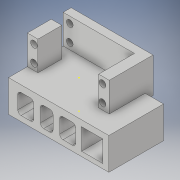
# Autodesk Inventor part: Nov 21 holder for arm server (resized hole)
Saved by Autodesk Inventor 2018 (Build 220112000, 112)
## iProperties
Created: 2017-11-08
Part Number: Nov 21 holder for arm server (resized hole)
Material: Generic
Document SubType Name: Modeling
Designer: battin.michael
Density: 1 g/cm^3
Appearance: Default
Author: battin.michael
Autodesk Inventor part; units mm, degrees
ref_plane "YZ Plane" through (0, 0, 0) normal (1, 0, 0) x (0, 1, 0)
ref_plane "XZ Plane" through (0, 0, 0) normal (0, 1, 0) x (-1, 0, 0)
ref_plane "XY Plane" through (0, 0, 0) normal (0, 0, 1) x (1, 0, 0)
sketch "Sketch1" plane through (0, 0, 0) normal (0, 1, 0) x (-1, 0, 0)
  line L0 (59.1344, 5.7229) -> (-34.3376, 5.7229)
  line L1 (-34.3376, 5.7229) -> (-34.3376, -46.6011)
  line L2 (-34.3376, -46.6011) -> (59.1344, -46.6011)
  line L3 (59.1344, -46.6011) -> (59.1344, 5.7229)
  point P0 (0, 0)
  dimension "d0" = 52.324
  dimension "d1" = 93.472
  constraints: 8 end point, 2 parallel, 1 horizontal, 1 perpendicular
  measures "d0" distance between parallel lines of L2 L0
  measures "d1" distance between parallel lines of L1 L3
extrude "Extrusion1" add sketch "Sketch1" along normal blind 5.08
sketch "Sketch2" plane through (0, 5.08, 0) normal (0, 1, 0) x (1, 0, 0)
  line L0 (34.3376, -5.7229) -> (34.3376, 46.6011) projected
  line L1 (-59.1344, -5.7229) -> (34.3376, -5.7229) projected
  line L2 (34.3376, 46.6011) -> (27.9876, 46.6011)
  line L3 (27.9876, 46.6011) -> (27.9876, -5.7229)
  line L4 (27.9876, -5.7229) -> (34.3376, -5.7229)
  line L5 (34.3376, -5.7229) -> (34.3376, 46.6011)
  line L6 (8.9376, 46.6011) -> (2.5876, 46.6011)
  line L7 (2.5876, 46.6011) -> (2.5876, -5.7229)
  line L8 (2.5876, -5.7229) -> (8.9376, -5.7229)
  line L9 (8.9376, -5.7229) -> (8.9376, 46.6011)
  line L10 (34.3376, 46.6011) -> (-59.1344, 46.6011) projected
  line L11 (-59.1344, 46.6011) -> (-59.1344, -5.7229) projected
  line L12 (-52.7844, 46.6011) -> (-59.1344, 46.6011)
  line L13 (-59.1344, 46.6011) -> (-59.1344, -5.7229)
  line L14 (-59.1344, -5.7229) -> (-52.7844, -5.7229)
  line L15 (-52.7844, -5.7229) -> (-52.7844, 46.6011)
  point P0 (0, 0)
  dimension "d4" = 6.35
  dimension "d5" = 19.05
  dimension "d6" = 6.35
  dimension "d7" = 6.35
  constraints: 24 end point, 6 parallel, 3 horizontal, 3 perpendicular, 3 point on line
  measures "d4" distance between parallel lines of L0 L3
  measures "d5" distance between parallel lines of L3 L9
  measures "d6" distance between parallel lines of L7 L9
  measures "d7" distance between parallel lines of L13 L15
extrude "Extrusion2" add sketch "Sketch2" along normal blind 19.05 contours L1 L3 L2 L0 | L1 L7 L6 L9 | L1 L11 L10 L15
sketch "Sketch3" plane through (0, 24.13, 0) normal (0, 1, 0) x (1, 0, 0)
  line L0 (34.3376, -5.7229) -> (34.3376, 46.6011) projected
  line L1 (-59.1344, 46.6011) -> (-59.1344, -5.7229) projected
  line L2 (34.3376, 46.6011) -> (-59.1344, 46.6011)
  line L3 (-59.1344, 46.6011) -> (-59.1344, -5.7229)
  line L4 (-59.1344, -5.7229) -> (34.3376, -5.7229)
  line L5 (34.3376, -5.7229) -> (34.3376, 46.6011)
  point P0 (0, 0)
  constraints: 8 end point, 2 parallel, 1 horizontal, 1 perpendicular
extrude "Extrusion3" add sketch "Sketch3" along normal blind 6.35
sketch "Sketch4" plane through (0, 30.48, 0) normal (0, 1, 0) x (1, 0, 0)
  point P0 (0, 0)
sketch "Sketch5" plane through (0, 30.48, 0) normal (0, 1, 0) x (1, 0, 0)
  line L0 (-59.1344, -5.7229) -> (34.3376, -5.7229) projected
  line L1 (-59.1344, -5.7229) -> (-51.5144, -5.7229)
  line L2 (-51.5144, -5.7229) -> (-51.5144, 46.6011)
  line L3 (-51.5144, 46.6011) -> (-59.1344, 46.6011)
  line L4 (-59.1344, 46.6011) -> (-59.1344, -5.7229)
  line L5 (-52.7844, -5.7229) -> (2.5876, -5.7229) projected
  line L6 (6.5246, -5.7229) -> (14.1446, -5.7229)
  line L7 (14.1446, -5.7229) -> (14.1446, 46.6011)
  line L8 (14.1446, 46.6011) -> (6.5246, 46.6011)
  line L9 (6.5246, 46.6011) -> (6.5246, -5.7229)
  point P0 (0, 0)
  dimension "d12" = 7.62
  dimension "d13" = 7.62
  dimension "d14" = 58.039
  constraints: 16 end point, 4 parallel, 2 horizontal, 2 perpendicular, 1 point on line
  measures "d12" distance of L3.end L2.end
  measures "d13" distance of L8.end L7.end
  measures "d14" distance between parallel lines of L9 L2
extrude "Extrusion4" add sketch "Sketch5" along normal blind 27.94
sketch "Sketch6" plane through (0, 58.42, 0) normal (0, 1, 0) x (1, 0, 0)
  point P0 (0, 0)
sketch "Sketch7" plane through (0, 58.42, 0) normal (0, 1, 0) x (1, 0, 0)
  line L0 (-59.1344, -5.7229) -> (-51.5144, -5.7229) projected
  line L1 (-51.5144, -5.7229) -> (-51.5144, 46.6011) projected
  line L2 (-59.1344, -5.7229) -> (-51.5144, -5.7229)
  line L3 (-51.5144, -5.7229) -> (-51.5144, 12.3111)
  line L4 (-51.5144, 12.3111) -> (-59.1344, 12.3111)
  line L5 (-59.1344, 12.3111) -> (-59.1344, -5.7229)
  line L6 (6.5246, -5.7229) -> (6.5246, 46.6011) projected
  line L7 (14.1446, -5.7229) -> (14.1446, 46.6011) projected
  line L8 (6.5246, -5.7229) -> (14.1446, -5.7229)
  line L9 (14.1446, -5.7229) -> (14.1446, 12.3111)
  line L10 (14.1446, 12.3111) -> (6.5246, 12.3111)
  line L11 (6.5246, 12.3111) -> (6.5246, -5.7229)
  point P0 (0, 0)
  dimension "d17" = 18.034
  constraints: 16 end point, 4 parallel, 2 horizontal, 2 perpendicular, 2 point on line
  measures "d17" distance between parallel lines of L4 L0
extrude "Extrusion5" cut sketch "Sketch7" against normal blind 27.94
sketch "Sketch8" plane through (0, 58.42, 0) normal (0, 1, 0) x (1, 0, 0)
  line L0 (34.3376, 46.6011) -> (-59.1344, 46.6011) projected
  line L1 (-51.5144, 46.6011) -> (-51.5144, 12.3111) projected
  line L2 (-59.1344, 46.6011) -> (-51.5144, 46.6011)
  line L3 (-51.5144, 46.6011) -> (-51.5144, 35.1711)
  line L4 (-51.5144, 35.1711) -> (-59.1344, 35.1711)
  line L5 (-59.1344, 35.1711) -> (-59.1344, 46.6011)
  point P0 (0, 0)
  dimension "d20" = 11.43
  constraints: 8 end point, 2 parallel, 1 horizontal, 1 perpendicular, 1 point on line
  measures "d20" distance between parallel lines of L4 L0
extrude "Extrusion6" cut sketch "Sketch8" against normal blind 27.94
sketch "Sketch9" plane through (34.3376, 0, -46.6011) normal (0, 0, -1) x (-1, 0, 0)
  line L0 (93.472, 30.48) -> (0, 30.48) projected
  line L1 (27.813, 30.48) -> (20.193, 30.48) projected
  line L2 (93.472, 30.48) -> (20.193, 30.48)
  line L3 (20.193, 30.48) -> (20.193, 24.13)
  line L4 (6.35, 24.13) -> (25.4, 24.13) projected
  line L5 (31.75, 24.13) -> (87.122, 24.13) projected
  line L6 (25.4, 24.13) -> (31.75, 24.13)
  line L7 (87.122, 5.08) -> (87.122, 24.13) projected
  line L8 (31.75, 24.13) -> (87.122, 24.13)
  line L9 (93.472, 0) -> (93.472, 30.48) projected
  line L10 (87.122, 24.13) -> (93.472, 24.13)
  point P0 (34.3376, 0)
  constraints: 10 end point, 3 point on line, 2 horizontal, 2 perpendicular
extrude "Extrusion7" add sketch "Sketch9" along normal blind 7.62
sketch "Sketch10" plane through (0, 30.48, 0) normal (0, 1, 0) x (1, 0, 0)
  line L0 (14.1446, 46.6011) -> (14.1446, 54.2211) projected
  line L1 (-59.1344, 54.2211) -> (14.1446, 54.2211) projected
  line L2 (14.1446, 46.6011) -> (-59.1344, 46.6011)
  line L3 (-59.1344, 46.6011) -> (-59.1344, 54.2211)
  line L4 (-59.1344, 54.2211) -> (14.1446, 54.2211)
  line L5 (14.1446, 54.2211) -> (14.1446, 46.6011)
  point P0 (0, 0)
  constraints: 8 end point, 2 parallel, 1 horizontal, 1 perpendicular
extrude "Extrusion8" add sketch "Sketch10" along normal blind 27.94
fillet "Fillet1" radius 3.175 4 edges at (2.5876, 5.08, -20.4391) (-52.7844, 5.08, -20.4391) (2.5876, 24.13, -20.4391) (-52.7844, 24.13, -20.4391)
sketch "Sketch11" plane through (-59.1344, 58.42, -12.3111) normal (0, 0, 1) x (1, 0, 0)
  point P0 (59.1344, -58.42)
sketch "Sketch12" plane through (-59.1344, 58.42, -12.3111) normal (0, 0, 1) x (1, 0, 0)
  circle A0 centre (3.81, -6.096) radius 2.54
  line L0 (0, 0) -> (7.62, 0) projected
  line L1 (0, -27.94) -> (0, 0) projected
  circle A1 centre (3.81, -21.844) radius 2.54
  line L2 (0, -27.94) -> (7.62, -27.94) projected
  circle A2 centre (69.469, -6.096) radius 2.54
  line L3 (65.659, 0) -> (73.279, 0) projected
  line L4 (73.279, 0) -> (73.279, -27.94) projected
  circle A3 centre (69.469, -21.844) radius 2.54
  line L5 (0, -27.94) -> (93.472, -27.94) projected
  point P0 (59.1344, -58.42)
  dimension "d29" = 6.096
  dimension "d30" = 3.81
  dimension "d31" = 5.08
  dimension "d32" = 5.08
  dimension "d33" = 3.81
  dimension "d34" = 6.096
  dimension "d35" = 5.08
  dimension "d36" = 6.096
  dimension "d37" = 3.81
  dimension "d38" = 5.08
  dimension "d39" = 3.81
  dimension "d40" = 6.096
  constraints: 4 centre point
  measures "d29" distance from line of L0 A0.centre
  measures "d30" distance from line of L1 A0.centre
  measures "d31" diameter of A0
  measures "d32" diameter of A1
  measures "d33" distance from line of A1.centre L1
  measures "d34" distance from line of L2 A1.centre
  measures "d35" diameter of A2
  measures "d36" distance from line of A2.centre L3
  measures "d37" distance from line of A2.centre L4
  measures "d38" diameter of A3
  measures "d39" distance from line of A3.centre L4
  measures "d40" distance from line of L5 A3.centre
hole "Hole1" at (-55.3244, 52.324, -12.3111) at (-55.3244, 36.576, -12.3111) at (10.3346, 52.324, -12.3111) at (10.3346, 36.576, -12.3111) direction (0, 0, -1) diameter 6.35 end through all
sketch "Sketch13" plane through (-59.1344, 0, -46.6011) normal (-1, 0, 0) x (0, 0, 1)
  line L0 (-7.62, 24.13) -> (-7.62, 58.42) projected
  line L1 (-7.62, 58.42) -> (-7.62, 24.13)
  line L2 (0, 24.13) -> (-7.62, 24.13) projected
  line L3 (-7.62, 24.13) -> (0, 24.13)
  line L4 (0, 0) -> (0, 24.13) projected
  line L5 (0, 24.13) -> (0, 0)
  line L6 (0, 0) -> (52.324, 0) projected
  line L7 (0, 0) -> (52.324, 0)
  line L8 (52.324, 0) -> (52.324, 30.48) projected
  line L9 (52.324, 0) -> (52.324, 30.48)
  line L10 (34.29, 30.48) -> (34.29, 58.42) projected
  line L11 (52.324, 30.48) -> (34.29, 30.48)
  line L12 (34.29, 30.48) -> (34.29, 58.42)
  line L13 (34.29, 58.42) -> (11.43, 58.42) projected
  line L14 (34.29, 58.42) -> (11.43, 58.42)
  line L15 (11.43, 30.48) -> (11.43, 58.42) projected
  line L16 (11.43, 58.42) -> (11.43, 30.48)
  line L17 (11.43, 30.48) -> (0, 30.48) projected
  line L18 (11.43, 30.48) -> (0, 30.48)
  line L19 (0, 30.48) -> (0, 58.42) projected
  line L20 (0, 30.48) -> (0, 58.42)
  line L21 (34.29, 58.42) -> (-7.62, 58.42) projected
  line L22 (0, 58.42) -> (-7.62, 58.42)
  point P0 (46.6011, 0)
  constraints: 24 end point, 6 collinear, 3 perpendicular, 1 horizontal, 1 vertical
extrude "Extrusion9" add sketch "Sketch13" along normal blind 2.54 contours L0 L21 L19 L17 L15 L13 L10 L11 L8 L6 L4 L2
sketch "Sketch14" plane through (14.1446, 24.13, -46.6011) normal (1, 0, 0) x (0, 0, -1)
  line L0 (-34.29, 34.29) -> (7.62, 34.29) projected
  line L1 (7.62, 0) -> (7.62, 34.29) projected
  line L2 (-34.29, 34.29) -> (7.62, 34.29)
  line L3 (7.62, 34.29) -> (7.62, 0)
  line L4 (7.62, 0) -> (-34.29, 0)
  line L5 (-34.29, 0) -> (-34.29, 34.29)
  line L6 (0, 0) -> (7.62, 0) projected
  line L7 (0, 6.35) -> (-34.29, 6.35) projected
  line L8 (0, 0) -> (-34.29, 0)
  line L9 (-34.29, 0) -> (-34.29, 6.35)
  line L10 (-34.29, 6.35) -> (0, 6.35)
  line L11 (0, 6.35) -> (0, 0)
  point P0 (-46.6011, -24.13)
  constraints: 16 end point, 4 parallel, 2 horizontal, 2 perpendicular
extrude "Extrusion10" add sketch "Sketch14" along normal blind 2.54 contours L0 L1 L4 L11 L7 L5
sketch "Sketch15" plane through (0, 5.08, 0) normal (0, 1, 0) x (1, 0, 0)
  point P0 (0, 0)
sketch "Sketch16" plane through (0, 5.08, 0) normal (0, 1, 0) x (1, 0, 0)
  line L0 (34.3376, 46.6011) -> (-61.6744, 46.6011) projected
  line L1 (-61.6744, -5.7229) -> (34.3376, -5.7229) projected
  line L2 (-37.502, 46.6011) -> (-31.152, 46.6011)
  line L3 (-31.152, 46.6011) -> (-31.152, -5.7229)
  line L4 (-31.152, -5.7229) -> (-37.502, -5.7229)
  line L5 (-37.502, -5.7229) -> (-37.502, 46.6011)
  line L6 (-19.0447, -5.7229) -> (-12.6947, -5.7229)
  line L7 (-12.6947, -5.7229) -> (-12.6947, 46.6011)
  line L8 (-12.6947, 46.6011) -> (-19.0447, 46.6011)
  line L9 (-19.0447, 46.6011) -> (-19.0447, -5.7229)
  line L10 (-49.6094, -5.7229) -> (-49.6094, 46.6011) projected
  point P0 (0, 0)
  dimension "d52" = 6.35
  dimension "d53" = 6.35
  dimension "d54" = 12.1073
  dimension "d55" = 12.1073
  constraints: 16 end point, 4 parallel, 4 point on line, 2 horizontal, 2 perpendicular
  measures "d52" distance between parallel lines of L3 L5
  measures "d53" distance between parallel lines of L7 L9
  measures "d54" distance between parallel lines of L10 L5
  measures "d55" distance between parallel lines of L9 L3
extrude "Extrusion11" add sketch "Sketch16" along normal blind 25.4 contours L7 L1 L9 L0 | L3 L1 L5 L0
fillet "Fillet2" radius 3.175 1 edges at (-37.502, 5.08, -20.4391)
fillet "Fillet3" radius 3.175 1 edges at (-19.0447, 5.08, -20.4391)
fillet "Fillet4" radius 3.175 1 edges at (-31.152, 24.13, -20.4391)
fillet "Fillet5" radius 3.175 1 edges at (-12.6947, 24.13, -20.4391)
fillet "Fillet6" radius 3.175 1 edges at (-12.6947, 5.08, -20.4391)
fillet "Fillet7" radius 3.175 1 edges at (-31.152, 5.08, -20.4391)
fillet "Fillet8" radius 3.175 1 edges at (-37.502, 24.13, -20.4391)
fillet "Fillet9" radius 3.175 1 edges at (-19.0447, 24.13, -20.4391)
sketch "Sketch17" plane through (27.9876, 5.08, -46.6011) normal (-1, 0, 0) x (0, 0, 1)
  line L0 (0, 19.05) -> (-7.62, 19.05) projected
  line L1 (52.324, 0) -> (0, 0) projected
  line L2 (0, 19.05) -> (52.324, 19.05)
  line L3 (52.324, 19.05) -> (52.324, 0)
  line L4 (52.324, 0) -> (0, 0)
  line L5 (0, 0) -> (0, 19.05)
  point P0 (46.6011, -5.08)
  constraints: 8 end point, 2 parallel, 1 horizontal, 1 perpendicular
extrude "Extrusion12" cut sketch "Sketch17" against normal blind 0.635
sketch "Sketch18" plane through (8.9376, 5.08, 5.7229) normal (1, 0, 0) x (0, 0, -1)
  line L0 (52.324, 15.875) -> (52.324, 19.05) projected
  line L1 (0, 0) -> (52.324, 0) projected
  line L2 (52.324, 19.05) -> (0, 19.05)
  line L3 (0, 19.05) -> (0, 0)
  line L4 (0, 0) -> (52.324, 0)
  line L5 (52.324, 0) -> (52.324, 19.05)
  point P0 (5.7229, -5.08)
  constraints: 8 end point, 2 parallel, 1 horizontal, 1 perpendicular
extrude "Extrusion13" cut sketch "Sketch18" against normal blind 0.635
sketch "Sketch19" plane through (0, 24.13, 0) normal (0, -1, 0) x (1, 0, 0)
  line L0 (28.6226, 5.7229) -> (28.6226, -46.6011) projected
  line L1 (-61.6744, 5.7229) -> (34.3376, 5.7229) projected
  line L2 (28.6226, -46.6011) -> (8.1284, -46.6011)
  line L3 (8.1284, -46.6011) -> (8.1284, 5.7229)
  line L4 (8.1284, 5.7229) -> (28.6226, 5.7229)
  line L5 (28.6226, 5.7229) -> (28.6226, -46.6011)
  point P0 (0, 0)
  constraints: 8 end point, 2 parallel, 1 horizontal, 1 perpendicular, 1 point on line
extrude "Extrusion14" cut sketch "Sketch19" against normal blind 0.635
sketch "Sketch20" plane through (0, 5.08, 0) normal (0, 1, 0) x (1, 0, 0)
  line L0 (28.6226, -5.7229) -> (28.6226, 46.6011) projected
  line L1 (16.6846, 46.6011) -> (8.3026, 46.6011) projected
  line L2 (28.6226, -5.7229) -> (8.3026, -5.7229)
  line L3 (8.3026, -5.7229) -> (8.3026, 46.6011)
  line L4 (8.3026, 46.6011) -> (28.6226, 46.6011)
  line L5 (28.6226, 46.6011) -> (28.6226, -5.7229)
  point P0 (0, 0)
  constraints: 8 end point, 2 parallel, 1 horizontal, 1 perpendicular
extrude "Extrusion15" cut sketch "Sketch20" against normal blind 0.635
sketch "Sketch21" plane through (0, 24.13, 0) normal (0, -1, 0) x (1, 0, 0)
  line L0 (16.6846, -46.6011) -> (16.6846, -54.2211) projected
  line L1 (-49.6094, -46.6011) -> (-61.6744, -46.6011) projected
  line L2 (16.6846, -54.2211) -> (-61.6744, -54.2211)
  line L3 (-61.6744, -54.2211) -> (-61.6744, -46.6011)
  line L4 (-61.6744, -46.6011) -> (16.6846, -46.6011)
  line L5 (16.6846, -46.6011) -> (16.6846, -54.2211)
  point P0 (0, 0)
  constraints: 8 end point, 2 parallel, 1 horizontal, 1 perpendicular
extrude "Extrusion16" cut sketch "Sketch21" against normal blind 0.635
body "Solid1"
